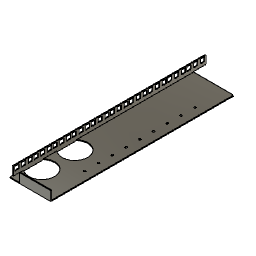
TV Cabinet Rack Posts (Autodesk Fusion 360 design; units mm, degrees)
Autodesk Fusion 360 part; units mm, degrees
sketch "Sketch4" plane through (0, -351, 0) normal (0, -1, 0) x (1, 0, 0)
  line L0 (-75, 0) -> (20, 0)
  line L1 (20, 0) -> (20, 2)
  line L2 (20, 2) -> (-73, 2)
  line L3 (-73, 2) -> (-73, 24.5)
  line L4 (-73, 24.5) -> (-75, 24.5)
  line L5 (-75, 24.5) -> (-75, 0)
  line L6 (20, 0) -> (-50, 0)
  line L7 (-50, 0) -> (-50, 24.5)
  line L8 (-50, 24.5) -> (20, 24.5)
  line L9 (20, 24.5) -> (20, 0)
  line L10 (-75, 0, -421) -> (-5, 0, -421)
  constraint horizontal L6
  constraint vertical L7
  constraint horizontal L8
  constraint vertical L9
  constraint coincident L0.end L1.start
  constraint equal L5 L7
sketch "Sketch1" plane through (0, 0, 0) normal (0, 0, 1) x (1, 0, 0) in component "Mock Rubber"
  circle A0 centre (0, 0) radius 5
  circle A1 centre (0, 0) radius 2.5
  dimension "d738" = 10
  dimension "d739" = 5
  constraint coincident A0.centre A1.centre
  constraint concentric A0 A1
  measures "d738" diameter of A0
  measures "d739" diameter of A1
extrude "Extrude1" add sketch "Sketch1" along normal blind 2 makes body 1 in component "Mock Rubber"
sketch "Sketch2" plane through (0, 0, 0) normal (0, 0, 1) x (1, 0, 0) in component "Mock Rubber"
  line L0 (65.4, 12.7) -> (40, 12.7)
  line L1 (40, 12.7) -> (40, -12.7)
  line L2 (40, -12.7) -> (65.4, -12.7)
  line L3 (65.4, -12.7) -> (65.4, 12.7)
  line L4 (65.4, 12.7) -> (40, -12.7) construction
  line L5 (40, 12.7) -> (65.4, -12.7) construction
  point P0 (52.7, 0)
  dimension "d745" = 25.4
  dimension "d746" = 25.4
  dimension "d747" = 40
  constraint horizontal L0
  constraint perpendicular L0 L1
  constraint parallel L0 L2
  constraint parallel L1 L3
  constraint coincident L4 P0
  constraint coincident L5 P0
  measures "d745" distance of L1.end L2.end
  measures "d746" distance of L0.end L1.end
  measures "d747" distance of origin L1
extrude "Extrude2" add sketch "Sketch2" along normal blind 4 separate body makes body 2 in component "Mock Rubber"
sketch "Sketch1 (2)" plane through (0, 0, 0) normal (0, 0, 1) x (1, 0, 0) in component "Rack Post"
  line L0 (-75, 70) -> (20, 70)
  line L1 (20, 70) -> (20, -355)
  line L2 (20, -355) -> (-75, -355)
  line L3 (-75, -355) -> (-75, 70)
  circle A0 centre (0, 0) radius 2.5
  circle A1 centre (0, -32) radius 2.5
  circle A2 centre (0, -64) radius 2.5
  circle A3 centre (0, -96) radius 2.5
  circle A4 centre (0, -128) radius 2.5
  circle A5 centre (0, -160) radius 2.5
  circle A6 centre (0, -192) radius 2.5
  circle A7 centre (0, -224) radius 2.5
  circle A8 centre (0, -256) radius 2.5
  circle A9 centre (-54, -225) radius 30
  circle A10 centre (-54, -302) radius 30
  dimension "d877" = 70
  dimension "d878" = 355
  dimension "d879" = 75
  dimension "d880" = 20
  dimension "d881" = 5
  dimension "d884" = 0
  dimension "d885" = -32
  dimension "d886" = 60
  dimension "d887" = 225
  dimension "d888" = 54
  dimension "d889" = 60
  dimension "d890" = 77
  dimension "d891" = 54
  constraint horizontal L0
  constraint vertical L1
  constraint horizontal L2
  constraint vertical L3
  constraint coincident A0.centre origin
  measures "d877" distance of A0.centre L0
  measures "d878" distance of A0.centre L2
  measures "d879" distance of A0.centre L3
  measures "d880" distance of A0.centre L1
  measures "d881" diameter of A0
  measures "d886" diameter of A9
  measures "d887" vertical distance of A0.centre A9.centre
  measures "d888" horizontal distance of A0.centre A9.centre
  measures "d889" diameter of A10
  measures "d890" vertical distance of A9.centre A10.centre
  measures "d891" horizontal distance of A0.centre A10.centre
extrude "Extrude1'" add sketch "Sketch1 (2)" along normal blind 2 separate body contours L0 L1 L2 L3 A9 A10 makes body 3 in component "Rack Post"
sketch "Sketch2 (2)" plane through (-75, 0, 0) normal (-1, 0, 0) x (0, -1, 0) in component "Rack Post"
  line L0 (-70, 0) -> (203.5757, 0)
  line L1 (203.5757, 0) -> (203.5757, 2)
  line L2 (203.5757, 2) -> (-70, 2)
  line L3 (-70, 2) -> (-70, 0)
  line L4 (-99, 0) -> (348.7, 0)
  line L5 (348.7, 0) -> (348.7, 22)
  line L6 (348.7, 22) -> (-99, 22)
  line L7 (-99, 22) -> (-99, 0)
  line L8 (-99, 0) -> (-70, 0)
  line L9 (-70, 0) -> (-70, 3)
  line L10 (-70, 3) -> (-99, 3)
  line L11 (-99, 3) -> (-99, 0)
  line L12 (-95.8, 19.75) -> (-86.3, 19.75)
  line L13 (-86.3, 19.75) -> (-86.3, 10.25)
  line L14 (-86.3, 10.25) -> (-95.8, 10.25)
  line L15 (-95.8, 10.25) -> (-95.8, 19.75)
  line L16 (-79.925, 10.25) -> (-79.925, 19.75)
  line L17 (-79.925, 19.75) -> (-70.425, 19.75)
  line L18 (-70.425, 10.25) -> (-79.925, 10.25)
  line L19 (-70.425, 19.75) -> (-70.425, 10.25)
  line L20 (-64.05, 10.25) -> (-64.05, 19.75)
  line L21 (-64.05, 19.75) -> (-54.55, 19.75)
  line L22 (-54.55, 10.25) -> (-64.05, 10.25)
  line L23 (-54.55, 19.75) -> (-54.55, 10.25)
  line L24 (-41.85, 10.25) -> (-51.35, 10.25)
  line L25 (-41.85, 19.75) -> (-41.85, 10.25)
  line L26 (-51.35, 19.75) -> (-41.85, 19.75)
  line L27 (-51.35, 10.25) -> (-51.35, 19.75)
  line L28 (-35.475, 10.25) -> (-35.475, 19.75)
  line L29 (-35.475, 19.75) -> (-25.975, 19.75)
  line L30 (-25.975, 19.75) -> (-25.975, 10.25)
  line L31 (-25.975, 10.25) -> (-35.475, 10.25)
  line L32 (-19.6, 10.25) -> (-19.6, 19.75)
  line L33 (-19.6, 19.75) -> (-10.1, 19.75)
  line L34 (-10.1, 19.75) -> (-10.1, 10.25)
  line L35 (-10.1, 10.25) -> (-19.6, 10.25)
  line L36 (2.6, 10.25) -> (-6.9, 10.25)
  line L37 (2.6, 19.75) -> (2.6, 10.25)
  line L38 (-6.9, 19.75) -> (2.6, 19.75)
  line L39 (-6.9, 10.25) -> (-6.9, 19.75)
  line L40 (8.975, 10.25) -> (8.975, 19.75)
  line L41 (8.975, 19.75) -> (18.475, 19.75)
  line L42 (18.475, 19.75) -> (18.475, 10.25)
  line L43 (18.475, 10.25) -> (8.975, 10.25)
  line L44 (24.85, 10.25) -> (24.85, 19.75)
  line L45 (24.85, 19.75) -> (34.35, 19.75)
  line L46 (34.35, 19.75) -> (34.35, 10.25)
  line L47 (34.35, 10.25) -> (24.85, 10.25)
  line L48 (47.05, 10.25) -> (37.55, 10.25)
  line L49 (47.05, 19.75) -> (47.05, 10.25)
  line L50 (37.55, 19.75) -> (47.05, 19.75)
  line L51 (37.55, 10.25) -> (37.55, 19.75)
  line L52 (53.425, 10.25) -> (53.425, 19.75)
  line L53 (53.425, 19.75) -> (62.925, 19.75)
  line L54 (62.925, 19.75) -> (62.925, 10.25)
  line L55 (62.925, 10.25) -> (53.425, 10.25)
  line L56 (69.3, 10.25) -> (69.3, 19.75)
  line L57 (69.3, 19.75) -> (78.8, 19.75)
  line L58 (78.8, 19.75) -> (78.8, 10.25)
  line L59 (78.8, 10.25) -> (69.3, 10.25)
  line L60 (91.5, 10.25) -> (82, 10.25)
  line L61 (91.5, 19.75) -> (91.5, 10.25)
  line L62 (82, 19.75) -> (91.5, 19.75)
  line L63 (82, 10.25) -> (82, 19.75)
  line L64 (97.875, 10.25) -> (97.875, 19.75)
  line L65 (97.875, 19.75) -> (107.375, 19.75)
  line L66 (107.375, 19.75) -> (107.375, 10.25)
  line L67 (107.375, 10.25) -> (97.875, 10.25)
  line L68 (113.75, 10.25) -> (113.75, 19.75)
  line L69 (113.75, 19.75) -> (123.25, 19.75)
  line L70 (123.25, 19.75) -> (123.25, 10.25)
  line L71 (123.25, 10.25) -> (113.75, 10.25)
  line L72 (135.95, 10.25) -> (126.45, 10.25)
  line L73 (135.95, 19.75) -> (135.95, 10.25)
  line L74 (126.45, 19.75) -> (135.95, 19.75)
  line L75 (126.45, 10.25) -> (126.45, 19.75)
  line L76 (142.325, 10.25) -> (142.325, 19.75)
  line L77 (142.325, 19.75) -> (151.825, 19.75)
  line L78 (151.825, 19.75) -> (151.825, 10.25)
  line L79 (151.825, 10.25) -> (142.325, 10.25)
  line L80 (158.2, 10.25) -> (158.2, 19.75)
  line L81 (158.2, 19.75) -> (167.7, 19.75)
  line L82 (167.7, 19.75) -> (167.7, 10.25)
  line L83 (167.7, 10.25) -> (158.2, 10.25)
  line L84 (180.4, 10.25) -> (170.9, 10.25)
  line L85 (180.4, 19.75) -> (180.4, 10.25)
  line L86 (170.9, 19.75) -> (180.4, 19.75)
  line L87 (170.9, 10.25) -> (170.9, 19.75)
  line L88 (186.775, 10.25) -> (186.775, 19.75)
  line L89 (186.775, 19.75) -> (196.275, 19.75)
  line L90 (196.275, 19.75) -> (196.275, 10.25)
  line L91 (196.275, 10.25) -> (186.775, 10.25)
  line L92 (202.65, 10.25) -> (202.65, 19.75)
  line L93 (202.65, 19.75) -> (212.15, 19.75)
  line L94 (212.15, 19.75) -> (212.15, 10.25)
  line L95 (212.15, 10.25) -> (202.65, 10.25)
  line L96 (224.85, 10.25) -> (215.35, 10.25)
  line L97 (224.85, 19.75) -> (224.85, 10.25)
  line L98 (215.35, 19.75) -> (224.85, 19.75)
  line L99 (215.35, 10.25) -> (215.35, 19.75)
  line L100 (231.225, 10.25) -> (231.225, 19.75)
  line L101 (231.225, 19.75) -> (240.725, 19.75)
  line L102 (240.725, 19.75) -> (240.725, 10.25)
  line L103 (240.725, 10.25) -> (231.225, 10.25)
  line L104 (247.1, 10.25) -> (247.1, 19.75)
  line L105 (247.1, 19.75) -> (256.6, 19.75)
  line L106 (256.6, 19.75) -> (256.6, 10.25)
  line L107 (256.6, 10.25) -> (247.1, 10.25)
  line L108 (269.3, 10.25) -> (259.8, 10.25)
  line L109 (269.3, 19.75) -> (269.3, 10.25)
  line L110 (259.8, 19.75) -> (269.3, 19.75)
  line L111 (259.8, 10.25) -> (259.8, 19.75)
  line L112 (275.675, 10.25) -> (275.675, 19.75)
  line L113 (275.675, 19.75) -> (285.175, 19.75)
  line L114 (285.175, 19.75) -> (285.175, 10.25)
  line L115 (285.175, 10.25) -> (275.675, 10.25)
  line L116 (291.55, 10.25) -> (291.55, 19.75)
  line L117 (291.55, 19.75) -> (301.05, 19.75)
  line L118 (301.05, 19.75) -> (301.05, 10.25)
  line L119 (301.05, 10.25) -> (291.55, 10.25)
  line L120 (313.75, 10.25) -> (304.25, 10.25)
  line L121 (313.75, 19.75) -> (313.75, 10.25)
  line L122 (304.25, 19.75) -> (313.75, 19.75)
  line L123 (304.25, 10.25) -> (304.25, 19.75)
  line L124 (320.125, 10.25) -> (320.125, 19.75)
  line L125 (320.125, 19.75) -> (329.625, 19.75)
  line L126 (329.625, 19.75) -> (329.625, 10.25)
  line L127 (329.625, 10.25) -> (320.125, 10.25)
  line L128 (336, 10.25) -> (336, 19.75)
  line L129 (336, 19.75) -> (345.5, 19.75)
  line L130 (345.5, 19.75) -> (345.5, 10.25)
  line L131 (345.5, 10.25) -> (336, 10.25)
  dimension "d894" = 22
  dimension "d895" = 447.7
  dimension "d896" = 99
  dimension "d897" = 70
  dimension "d898" = 3
  dimension "d899" = 9.5
  dimension "d900" = 9.5
  dimension "d901" = 2.25
  dimension "d902" = 3.2
  dimension "d905" = 15.875
  dimension "d906" = 0
  dimension "d909" = 44.45
  dimension "d910" = 0
  constraint horizontal L4
  constraint vertical L5
  constraint horizontal L6
  constraint vertical L7
  constraint coincident L0 L4.start
  constraint horizontal L8
  constraint vertical L9
  constraint horizontal L10
  constraint vertical L11
  constraint horizontal L12
  constraint vertical L13
  constraint horizontal L14
  constraint vertical L15
  measures "d894" distance of L4 L6
  measures "d895" distance of L5 L7
  measures "d896" distance of origin L7
  measures "d897" distance of origin L9
  measures "d898" distance of L4 L10
  measures "d899" distance of L12.start L12.end
  measures "d900" distance of L12.start L14.end
  measures "d901" distance of L6 L12
  measures "d902" distance of L7 L15
extrude "Extrude2'" add sketch "Sketch2 (2)" against normal blind 2 contours L0 L1 L2 L3 L4 L9 | L1 L2 L4 L5 L6 L7 L9 L10 bodies 3 in component "Rack Post"
sketch "Sketch3" plane through (0, -355, 0) normal (0, -1, 0) x (1, 0, 0) in component "Rack Post"
  line L0 (-75, 0) -> (20, 0)
  line L1 (20, 0) -> (20, 2)
  line L2 (20, 2) -> (-75, 2)
  line L3 (-75, 2) -> (-75, 0)
  line L4 (20, 0) -> (-53, 0)
  line L5 (-53, 0) -> (-53, 22)
  line L6 (-53, 22) -> (20, 22)
  line L7 (20, 22) -> (20, 0)
  line L8 (-73, 22) -> (-73, 2)
  dimension "d913" = 20
  dimension "d914" = 22
  constraint horizontal L4
  constraint vertical L5
  constraint horizontal L6
  constraint vertical L7
  constraint coincident L0.end L1.start
  measures "d913" distance of L5 L8
  measures "d914" distance of origin L6
extrude "Extrude3" add sketch "Sketch3" against normal blind 2 contours L2 L5 L6 L7 bodies 3 in component "Rack Post"
sketch "Sketch6" plane through (0, 0, 0) normal (0, 0, 1) x (1, 0, 0)
  line L0 (-101.6255, -68.5) -> (87.4947, -68.5)
  line L1 (97.3995, -179) -> (-116.9977, -179)
  point P0 (20, 97)
  point P1 (-75, -351)
  dimension "d450" = 165.5
  dimension "d451" = 172
  constraint horizontal L0
  constraint horizontal L1
  measures "d450" vertical distance of L0.end P0
  measures "d451" vertical distance of L1.end P1
sketch "Sketch1 (3)" plane through (0, 0, 0) normal (0, 0, 1) x (1, 0, 0) in component "Door Stop"
  line L0 (-15, 10) -> (19, 10)
  line L1 (19, 10) -> (19, -9)
  line L2 (19, -9) -> (-15, -9)
  line L3 (-15, -9) -> (-15, 10)
  dimension "d544" = 19
  dimension "d545" = 9
  dimension "d546" = 10
  dimension "d547" = 15
  constraint horizontal L0
  constraint vertical L1
  constraint horizontal L2
  constraint vertical L3
  measures "d544" distance of origin L1
  measures "d545" distance of origin L2
  measures "d546" distance of origin L0
  measures "d547" distance of origin L3
extrude "Extrude1''" [rolled back] along distance 1.5 taper angle 0 in component "Door Stop"
sketch "Sketch2 (3)" plane through (0, 0, 1.5) normal (0, 0, 1) x (-1, 0, 0) in component "Door Stop"
  line L0 (15, 9) -> (-19, 9)
  line L1 (-19, 9) -> (-19, -10)
  line L2 (-19, -10) -> (15, -10)
  line L3 (15, -10) -> (15, 9)
  circle A0 centre (0, 0) radius 2
  dimension "d550" = 4
  constraint coincident A0.centre origin
  measures "d550" diameter of A0
extrude "Extrude2''" [rolled back] side1offset 0 taper angle 0 in component "Door Stop"
sketch "Sketch3 (2)" plane through (0, 0, 1.5) normal (0, 0, 1) x (-1, 0, 0) in component "Door Stop"
  circle A0 centre (0, 0) radius 2
  line L0 (15, 9) -> (-19, 9)
  line L1 (-19, 9) -> (-19, -10)
  line L2 (-19, -10) -> (15, -10)
  line L3 (15, -10) -> (15, 9)
  line L4 (-19, 9) -> (-17, 9)
  line L5 (-17, 9) -> (-17, -10)
  line L6 (-17, -10) -> (-19, -10)
  line L7 (-19, -10) -> (-19, 9)
  dimension "d553" = 2
  constraint horizontal L4
  constraint vertical L5
  constraint horizontal L6
  constraint vertical L7
  constraint coincident L2 L5.end
  constraint coincident L0.end L1.start
  measures "d553" distance of L5 L7
extrude "Extrude3'" [rolled back] along distance 8 taper angle 0 in component "Door Stop"
sketch "Sketch4 (2)" plane through (0, -9, 0) normal (0, -1, 0) x (1, 0, 0) in component "Door Stop"
  line L0 (-15, 0) -> (19, 0)
  line L1 (19, 0) -> (19, 9.5)
  line L2 (19, 9.5) -> (17, 9.5)
  line L3 (17, 9.5) -> (17, 1.5)
  line L4 (17, 1.5) -> (-15, 1.5)
  line L5 (-15, 1.5) -> (-15, 0)
  line L6 (17, 9.5) -> (-15, 1.5)
  constraint coincident L2.end L3.start
  constraint coincident L4.end L5.start
extrude "Extrude4" [rolled back] along distance -2 taper angle 0 in component "Door Stop"
sketch "Sketch5" plane through (0, 0, 0) normal (0, 0, 1) x (1, 0, 0) in component "Door Stop"
  line L0 (-2.9829, 0.5) -> (40.9829, 0.5) construction
  line L1 (19, 10) -> (19, -9) construction
  constraint midpoint L0 L1
sketch "Sketch6 (2)" plane through (0, 10, 0) normal (0, 1, 0) x (-1, 0, 0) in component "Door Stop"
  line L0 (-19, 0) -> (15, 0)
  line L1 (15, 0) -> (15, 1.5)
  line L2 (15, 1.5) -> (-17, 1.5)
  line L3 (-17, 1.5) -> (-17, 9.5)
  line L4 (-17, 9.5) -> (-19, 9.5)
  line L5 (-19, 9.5) -> (-19, 0)
  line L6 (-17, 9.5) -> (15, 1.5)
  constraint coincident L3.end L4.start
  constraint coincident L1.end L2.start
extrude "Extrude5" [rolled back] along distance -2 taper angle 0 in component "Door Stop"
component "Mock Rubber" placed x (1, 0, 0) y (0, 1, 0) z (0, 0, 1) at (0, 0, 0)
component "Rack Post" placed x (1, 0, 0) y (0, 1, 0) z (0, 0, 1) at (0, 0, 0)
